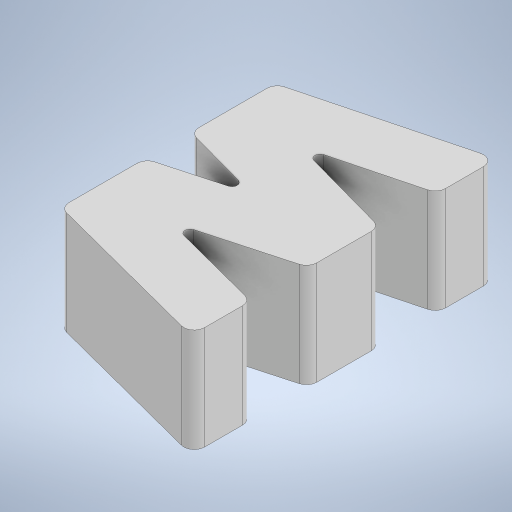
# Autodesk Inventor part: modulo_real
Saved by Autodesk Inventor 2023 (Build 270158000, 158)
## iProperties
Created: 2024-03-05
Part Number: modulo_real
Material: Genérico
Document SubType Name: Modeling
Designer: juana
Density: 1 g/cm^3
Appearance: Valor por defecto
Author: juana
Autodesk Inventor part; units mm, degrees
ref_plane "YZ Plane" through (0, 0, 0) normal (1, 0, 0) x (0, 1, 0)
ref_plane "XZ Plane" through (0, 0, 0) normal (0, 1, 0) x (-1, 0, 0)
ref_plane "XY Plane" through (0, 0, 0) normal (0, 0, 1) x (1, 0, 0)
sketch "Boceto1" plane through (0, 0, 0) normal (0, 1, 0) x (-1, 0, 0)
  line L0 (22.124, -21.4137) -> (22.124, -29.9725)
  line L1 (0, -35.058) -> (0, -30.2797)
  line L2 (0, -20.951) -> (0, -14.1069)
  line L3 (0, -4.7783) -> (0, 0)
  arc A0 (11.3452, -9.9915) -> (11.3364, -8.7359) centre (11.1725, -9.3649) ccw
  arc A1 (11.3364, -26.3221) -> (11.3452, -25.0664) centre (11.1725, -25.6931) ccw
  arc A2 (13.8914, -16.9023) -> (13.8914, -18.1556) centre (14.064, -17.529) ccw
  line L4 (22.124, -13.6443) -> (22.124, -5.0855)
  arc A3 (21.1517, -31.2305) -> (22.124, -29.9725) centre (20.824, -29.9725) ccw
  arc A4 (22.124, -5.0855) -> (21.1517, -3.8275) centre (20.824, -5.0855) ccw
  line L5 (13.8914, -16.9023) -> (21.1692, -14.8976)
  line L6 (13.8914, -18.1556) -> (21.1692, -20.1603)
  arc A5 (21.1692, -14.8976) -> (22.124, -13.6443) centre (20.824, -13.6443) ccw
  arc A6 (22.124, -21.4137) -> (21.1692, -20.1603) centre (20.824, -21.4137) ccw
  arc A7 (0, -35.058) -> (1.6277, -36.316) centre (1.3, -35.058) ccw
  line L7 (21.1517, -3.8275) -> (1.6277, 1.258)
  arc A8 (1.6277, 1.258) -> (0, 0) centre (1.3, 0) ccw
  line L8 (11.3364, -8.7359) -> (0.9723, -6.0363)
  arc A9 (0, -4.7783) -> (0.9723, -6.0363) centre (1.3, -4.7783) ccw
  line L9 (11.3452, -9.9915) -> (0.9548, -12.8536)
  arc A10 (0.9548, -12.8536) -> (0, -14.1069) centre (1.3, -14.1069) ccw
  arc A11 (0, -20.951) -> (0.9548, -22.2043) centre (1.3, -20.951) ccw
  line L10 (0.9548, -22.2043) -> (11.3452, -25.0664)
  line L11 (11.3364, -26.3221) -> (0.9723, -29.0217)
  arc A12 (0.9723, -29.0217) -> (0, -30.2797) centre (1.3, -30.2797) ccw
  line L12 (22.124, -5.0855) -> (22.124, -29.9725) construction
  line L13 (21.1517, -31.2305) -> (1.6277, -36.316)
  point P0 (13.414, -17.529)
  point P1 (11.8225, -25.6976)
  point P2 (22.124, -17.529)
  point P3 (0, -17.529)
  point P4 (22.124, -9.3649)
  point P5 (22.124, -25.6931)
  dimension "d17" = 0.65
  dimension "d41" = 1.3
  dimension "d42" = 30
  dimension "d43" = 30
  dimension "d44" = 7.224
  dimension "d47" = 24.887
  dimension "d48" = 22.124
  dimension "d50" = 8.661
  dimension "d51" = 14.064
  constraints: 28 end point, 28 point on circle, 26 tangent, 13 centre point, 11 equal radius, 5 parallel, 5 vertical, 4 horizontal alignment, 4 midpoint, 4 vertical alignment, 2 collinear
  measures "d17" radius of A2
  measures "d41" radius of A4
  measures "d42" angle of L8 L9
  measures "d43" angle of L10 L11
  measures "d44" distance between parallel lines of L8 L7
  measures "d47" distance of A4.centre A3.centre
  measures "d48" distance between parallel lines of L2 L12
  measures "d50" distance of A2.centre A1.centre
  measures "d51" distance of point (0, -17.529) A2.centre
extrude "Extrusión1" add sketch "Boceto1" along normal blind 13
sketch "Boceto2" plane through (0, 13, 0) normal (0, 1, 0) x (1, 0, 0)
  arc A0 (-21.1692, 14.8976) -> (-22.124, 13.6443) centre (-20.824, 13.6443) ccw projected
  line L0 (-22.124, 13.6443) -> (-22.124, 5.0855) projected
  arc A1 (-22.124, 5.0855) -> (-21.1517, 3.8275) centre (-20.824, 5.0855) ccw projected
  line L1 (-21.1517, 3.8275) -> (-1.6277, -1.258) projected
  arc A2 (-1.6277, -1.258) -> (0, 0) centre (-1.3, 0) ccw projected
  line L2 (0, 0) -> (0, 4.7783) projected
  arc A3 (0, 4.7783) -> (-0.9723, 6.0363) centre (-1.3, 4.7783) ccw projected
  line L3 (-0.9723, 6.0363) -> (-11.3364, 8.7359) projected
  arc A4 (-11.3452, 9.9915) -> (-11.3364, 8.7359) centre (-11.1725, 9.3649) ccw projected
  line L4 (-11.3452, 9.9915) -> (-0.9548, 12.8536) projected
  arc A5 (-0.9548, 12.8536) -> (0, 14.1069) centre (-1.3, 14.1069) ccw projected
  line L5 (0, 14.1069) -> (0, 20.951) projected
  arc A6 (0, 20.951) -> (-0.9548, 22.2043) centre (-1.3, 20.951) ccw projected
  line L6 (-0.9548, 22.2043) -> (-11.3452, 25.0664) projected
  arc A7 (-11.3364, 26.3221) -> (-11.3452, 25.0664) centre (-11.1725, 25.6931) ccw projected
  line L7 (-11.3364, 26.3221) -> (-0.9723, 29.0217) projected
  arc A8 (-0.9723, 29.0217) -> (0, 30.2797) centre (-1.3, 30.2797) ccw projected
  line L8 (0, 30.2797) -> (0, 35.058) projected
  arc A9 (0, 35.058) -> (-1.6277, 36.316) centre (-1.3, 35.058) ccw projected
  line L9 (-1.6277, 36.316) -> (-21.1517, 31.2305) projected
  arc A10 (-21.1517, 31.2305) -> (-22.124, 29.9725) centre (-20.824, 29.9725) ccw projected
  line L10 (-22.124, 29.9725) -> (-22.124, 21.4137) projected
  arc A11 (-22.124, 21.4137) -> (-21.1692, 20.1603) centre (-20.824, 21.4137) ccw projected
  line L11 (-21.1692, 20.1603) -> (-13.8914, 18.1556) projected
  arc A12 (-13.8914, 16.9023) -> (-13.8914, 18.1556) centre (-14.064, 17.529) ccw projected
  line L12 (-13.8914, 16.9023) -> (-21.1692, 14.8976) projected
  line L13 (-20.924, 5.0855) -> (-20.924, 13.6443)
  arc A13 (-20.8506, 13.7407) -> (-20.924, 13.6443) centre (-20.824, 13.6443) ccw
  line L14 (-20.8506, 13.7407) -> (-13.5727, 15.7454)
  arc A14 (-13.5727, 15.7454) -> (-13.5727, 19.3126) centre (-14.064, 17.529) ccw
  line L15 (-13.5727, 19.3126) -> (-20.8506, 21.3173)
  arc A15 (-20.924, 21.4137) -> (-20.8506, 21.3173) centre (-20.824, 21.4137) ccw
  line L16 (-20.924, 21.4137) -> (-20.924, 29.9725)
  arc A16 (-20.8492, 30.0693) -> (-20.924, 29.9725) centre (-20.824, 29.9725) ccw
  line L17 (-20.8492, 30.0693) -> (-1.3252, 35.1547)
  arc A17 (-1.2, 35.058) -> (-1.3252, 35.1547) centre (-1.3, 35.058) ccw
  line L18 (-1.2, 35.058) -> (-1.2, 30.2797)
  arc A18 (-1.2748, 30.1829) -> (-1.2, 30.2797) centre (-1.3, 30.2797) ccw
  line L19 (-1.2748, 30.1829) -> (-11.6389, 27.4833)
  arc A19 (-11.6389, 27.4833) -> (-11.6638, 23.9095) centre (-11.1725, 25.6931) ccw
  line L20 (-11.6638, 23.9095) -> (-1.2734, 21.0474)
  arc A20 (-1.2, 20.951) -> (-1.2734, 21.0474) centre (-1.3, 20.951) ccw
  line L21 (-1.2, 20.951) -> (-1.2, 14.1069)
  arc A21 (-1.2734, 14.0105) -> (-1.2, 14.1069) centre (-1.3, 14.1069) ccw
  line L22 (-1.2734, 14.0105) -> (-11.6638, 11.1485)
  arc A22 (-11.6638, 11.1485) -> (-11.6389, 7.5746) centre (-11.1725, 9.3649) ccw
  line L23 (-11.6389, 7.5746) -> (-1.2748, 4.8751)
  arc A23 (-1.2, 4.7783) -> (-1.2748, 4.8751) centre (-1.3, 4.7783) ccw
  line L24 (-1.2, 4.7783) -> (-1.2, 0)
  arc A24 (-1.3252, -0.0968) -> (-1.2, 0) centre (-1.3, 0) ccw
  line L25 (-1.3252, -0.0968) -> (-20.8492, 4.9887)
  arc A25 (-20.924, 5.0855) -> (-20.8492, 4.9887) centre (-20.824, 5.0855) ccw
  dimension "d52" = 1.2
  constraints: 26 end point, 26 point on circle, 13 centre point, 25 other
  measures "d52" distance between parallel lines of L0 L13
extrude "Extrusión2" add sketch "Boceto2" against normal blind 13 separate body contours L13 A13 L14 A14 L15 A15 L16 A16 L17 A17 L18 A18 L19 A19 L20 A20 L21 A21 L22 A22 L23 A23 L24 A24 L25 A25
sketch "Boceto3" plane through (0, 0, 0) normal (0, -1, 0) x (1, 0, 0)
  line L0 (-1.2, -4.7783) -> (-1.2, 0) projected
  arc A0 (-1.2, 0) -> (-1.3252, 0.0968) centre (-1.3, 0) ccw projected
  line L1 (-1.3252, 0.0968) -> (-20.8492, -4.9887) projected
  arc A1 (-20.8492, -4.9887) -> (-20.924, -5.0855) centre (-20.824, -5.0855) ccw projected
  line L2 (-20.924, -5.0855) -> (-20.924, -13.6443) projected
  arc A2 (-20.924, -13.6443) -> (-20.8506, -13.7407) centre (-20.824, -13.6443) ccw projected
  line L3 (-20.8506, -13.7407) -> (-13.5727, -15.7454) projected
  arc A3 (-13.5727, -19.3126) -> (-13.5727, -15.7454) centre (-14.064, -17.529) ccw projected
  line L4 (-13.5727, -19.3126) -> (-20.8506, -21.3173) projected
  arc A4 (-20.8506, -21.3173) -> (-20.924, -21.4137) centre (-20.824, -21.4137) ccw projected
  line L5 (-20.924, -21.4137) -> (-20.924, -29.9725) projected
  arc A5 (-20.924, -29.9725) -> (-20.8492, -30.0693) centre (-20.824, -29.9725) ccw projected
  line L6 (-20.8492, -30.0693) -> (-1.3252, -35.1547) projected
  arc A6 (-1.3252, -35.1547) -> (-1.2, -35.058) centre (-1.3, -35.058) ccw projected
  line L7 (-1.2, -35.058) -> (-1.2, -30.2797) projected
  arc A7 (-1.2, -30.2797) -> (-1.2748, -30.1829) centre (-1.3, -30.2797) ccw projected
  line L8 (-1.2748, -30.1829) -> (-11.6389, -27.4833) projected
  arc A8 (-11.6638, -23.9095) -> (-11.6389, -27.4833) centre (-11.1725, -25.6931) ccw projected
  line L9 (-11.6638, -23.9095) -> (-1.2734, -21.0474) projected
  arc A9 (-1.2734, -21.0474) -> (-1.2, -20.951) centre (-1.3, -20.951) ccw projected
  line L10 (-1.2, -20.951) -> (-1.2, -14.1069) projected
  arc A10 (-1.2, -14.1069) -> (-1.2734, -14.0105) centre (-1.3, -14.1069) ccw projected
  line L11 (-1.2734, -14.0105) -> (-11.6638, -11.1485) projected
  arc A11 (-11.6389, -7.5746) -> (-11.6638, -11.1485) centre (-11.1725, -9.3649) ccw projected
  line L12 (-11.6389, -7.5746) -> (-1.2748, -4.8751) projected
  arc A12 (-1.2748, -4.8751) -> (-1.2, -4.7783) centre (-1.3, -4.7783) ccw projected
  point P0 (0, 0)
extrude "Extrusión3" cut sketch "Boceto3" against normal blind 1.2 bodies 2
sketch "Boceto4" plane through (0, 13, 0) normal (0, 1, 0) x (1, 0, 0)
  line L0 (-1.2, 0) -> (-1.2, 4.7783) projected
  arc A0 (-1.2, 4.7783) -> (-1.2748, 4.8751) centre (-1.3, 4.7783) ccw projected
  line L1 (-1.2748, 4.8751) -> (-11.6389, 7.5746) projected
  arc A1 (-11.6638, 11.1485) -> (-11.6389, 7.5746) centre (-11.1725, 9.3649) ccw projected
  line L2 (-11.6638, 11.1485) -> (-1.2734, 14.0105) projected
  arc A2 (-1.2734, 14.0105) -> (-1.2, 14.1069) centre (-1.3, 14.1069) ccw projected
  line L3 (-1.2, 14.1069) -> (-1.2, 20.951) projected
  arc A3 (-1.2, 20.951) -> (-1.2734, 21.0474) centre (-1.3, 20.951) ccw projected
  line L4 (-1.2734, 21.0474) -> (-11.6638, 23.9095) projected
  arc A4 (-11.6389, 27.4833) -> (-11.6638, 23.9095) centre (-11.1725, 25.6931) ccw projected
  line L5 (-11.6389, 27.4833) -> (-1.2748, 30.1829) projected
  arc A5 (-1.2748, 30.1829) -> (-1.2, 30.2797) centre (-1.3, 30.2797) ccw projected
  line L6 (-1.2, 30.2797) -> (-1.2, 35.058) projected
  arc A6 (-1.2, 35.058) -> (-1.3252, 35.1547) centre (-1.3, 35.058) ccw projected
  line L7 (-1.3252, 35.1547) -> (-20.8492, 30.0693) projected
  arc A7 (-20.8492, 30.0693) -> (-20.924, 29.9725) centre (-20.824, 29.9725) ccw projected
  line L8 (-20.924, 29.9725) -> (-20.924, 21.4137) projected
  arc A8 (-20.924, 21.4137) -> (-20.8506, 21.3173) centre (-20.824, 21.4137) ccw projected
  line L9 (-20.8506, 21.3173) -> (-13.5727, 19.3126) projected
  arc A9 (-13.5727, 15.7454) -> (-13.5727, 19.3126) centre (-14.064, 17.529) ccw projected
  line L10 (-13.5727, 15.7454) -> (-20.8506, 13.7407) projected
  arc A10 (-20.8506, 13.7407) -> (-20.924, 13.6443) centre (-20.824, 13.6443) ccw projected
  line L11 (-20.924, 13.6443) -> (-20.924, 5.0855) projected
  arc A11 (-20.924, 5.0855) -> (-20.8492, 4.9887) centre (-20.824, 5.0855) ccw projected
  line L12 (-20.8492, 4.9887) -> (-1.3252, -0.0968) projected
  arc A12 (-1.3252, -0.0968) -> (-1.2, 0) centre (-1.3, 0) ccw projected
  point P0 (0, 0)
extrude "Extrusión4" cut sketch "Boceto4" against normal blind 1.2 bodies 2
equation "\"grosor_delgado\" = 1.2"
equation "\"grosor_grueso\" = 3.4"
